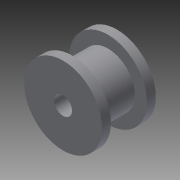
# Autodesk Inventor part: IdlePulley
Saved by Autodesk Inventor 2015 (Build 190159000, 159)
## iProperties
Created: 2017-01-05
Part Number: IdlePulley
Material: Generic
Document SubType Name: Modeling
Designer: Ernest
Density: 1 g/cm^3
Appearance: Default
Mass: 0.716283 g
Surface Area: 7.66549 cm^2
Volume: 0.716283 cm^3
Author: Ernest
Autodesk Inventor part; units mm, degrees
ref_plane "YZ Plane" through (0, 0, 0) normal (1, 0, 0) x (0, 1, 0)
ref_plane "XZ Plane" through (0, 0, 0) normal (0, 1, 0) x (-1, 0, 0)
ref_plane "XY Plane" through (0, 0, 0) normal (0, 0, 1) x (1, 0, 0)
sketch "Sketch1" plane through (0, 0, 0) normal (0, 0, 1) x (1, 0, 0)
  line L0 (1.5, 0) -> (1.5, 9)
  line L1 (1.5, 9) -> (6.5, 9)
  line L2 (6.5, 9) -> (6.5, 7.5)
  line L3 (6.5, 7.5) -> (4.5, 7.5)
  line L4 (4.5, 7.5) -> (4.5, 1.5)
  line L5 (4.5, 1.5) -> (6.5, 1.5)
  line L6 (6.5, 1.5) -> (6.5, 0)
  line L7 (6.5, 0) -> (1.5, 0)
  line L8 (0, -1.8) -> (0, 10.8) projected
  point P0 (0, 0)
  dimension "d0" = 9
  dimension "d1" = 5
  dimension "d2" = 1.5
  dimension "d3" = 2
  dimension "d4" = 1.5
  constraints: 16 end point, 6 perpendicular, 3 point on line, 1 collinear, 1 vertical
  measures "d0" distance of L0.start L0.end
  measures "d1" distance of L0.end L1.end
  measures "d2" distance of L1.end L2.end
  measures "d3" distance of L2.end L3.end
  measures "d4" distance from line of L0 point (0, 0)
revolve "Revolution1" add sketch "Sketch1" angle 360 about axis through (0, -10, 0) along (0, 1, 0)
body "Solid1"
